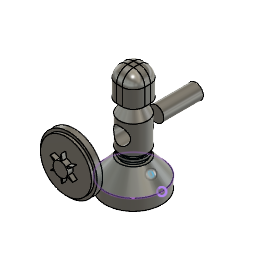
chess- pawn (Autodesk Fusion 360 design; units mm, degrees)
part number: 2026-07-03-03-44-02-403
Autodesk Fusion 360 part; units mm, degrees
sketch "Sketch1" plane through (0, 0, 0) normal (0, 0, 1) x (1, 0, 0)
  line L0 (0, 0) -> (12.7, 0)
  line L1 (12.7, 0) -> (12.7, 5.08)
  line L2 (12.7, 5.08) -> (6.35, 12.8383)
  line L3 (6.35, 12.8383) -> (5.08, 12.8383)
  line L4 (5.08, 12.8383) -> (5.08, 14.1186)
  line L5 (5.08, 14.1186) -> (5.715, 14.1186)
  line L6 (5.715, 14.1186) -> (5.715, 15.24)
  line L7 (5.715, 15.24) -> (5.08, 15.24)
  line L8 (5.08, 15.24) -> (5.08, 16.7432)
  line L9 (5.08, 16.7432) -> (6.35, 16.7432)
  line L10 (6.35, 16.7432) -> (6.35, 29.4432)
  line L11 (6.35, 29.4432) -> (2.54, 35.56)
  line L12 (2.54, 35.56) -> (0, 35.56)
  line L13 (0, 35.56) -> (0, 0)
  dimension "d1" = 12.7
  constraint coincident L0.start L13.end
  constraint horizontal L0
  constraint perpendicular L0 L1
  constraint perpendicular L1 L3
  constraint perpendicular L3 L4
  constraint perpendicular L4 L5
  constraint perpendicular L3 L6
  constraint perpendicular L6 L7
  constraint perpendicular L7 L8
  constraint perpendicular L8 L9
  constraint perpendicular L9 L10
  constraint perpendicular L10 L12
  constraint perpendicular L0 L13
  measures "d1" distance of L9.end L10.end
revolve "Revolve1" add sketch "Sketch1" angle 360 about axis through (0, 35.56, 0) along (0, -1, 0) makes body 1
sketch "Sketch2" plane through (0, 0, 0) normal (0, 0, 1) x (1, 0, 0)
ref_plane "WorkPlane1" through (0, 0, 7.62) normal (0, 0, 1) x (1, 0, 0)
sketch "Sketch3" plane through (0, 0, 7.62) normal (0, 0, 1) x (1, 0, 0)
  circle A0 centre (38.7313, 11.9967) radius 12.7
  dimension "d4" = 25.4
  measures "d4" diameter of A0
extrude "Extrude1" add sketch "Sketch3" along normal blind 2.54 separate body makes body 2
sketch "Sketch4" plane through (0, 0, 10.16) normal (0, 0, 1) x (1, 0, 0)
  circle A0 centre (38.7313, 11.9967) radius 12.7
  circle A1 centre (38.7313, 11.9967) radius 11.43
  dimension "d7" = 22.86
  constraint concentric A0 A1
  measures "d7" diameter of A1
extrude "Extrude2" add sketch "Sketch4" along normal blind 1.27 contours A1 bodies 2
sketch "Sketch5" plane through (0, 0, 11.43) normal (0, 0, 1) x (1, 0, 0)
  circle A0 centre (38.7313, 11.9967) radius 11.43
  circle A1 centre (38.7313, 11.9967) radius 3.2108
  line L0 (37.976, 15.1174) -> (38.638, 17.1526)
  line L1 (38.638, 17.1526) -> (39.2641, 15.163)
  constraint concentric A0 A1
  constraint coincident A1 L0.start
  constraint coincident A1 L1.end
extrude "Extrude3" add sketch "Sketch5" along normal blind 2.54 contours A1 bodies 2
sketch "Sketch6" plane through (0, 0, 11.43) normal (0, 0, 1) x (1, 0, 0)
  circle A0 centre (38.7313, 11.9967) radius 3.2108
  circle A1 centre (38.7313, 11.9967) radius 11.43
  line L0 (38.1005, 15.145) -> (38.5764, 17.7658)
  line L1 (38.5764, 17.7658) -> (39.0696, 15.1896)
  arc A2 (39.0696, 15.1896) -> (38.1005, 15.145) centre (38.7313, 11.9967) ccw
  constraint coincident A0 L0.start
  constraint coincident A0 L1.end
extrude "Extrude4" add sketch "Sketch6" along normal blind 2.032 contours A0 L0 L1 A2 bodies 2
pattern_circular "C-Pattern1" count 6 over 360 about axis through (38.7313, 11.9967, 13.97) along (0, 0, 1) of "Extrude4"
hole "Hole1" at (0, 23.5919, 6.35) direction (0, 0, -1) diameter 7.62 depth 12.7 tip angle 118 bodies 1
sketch "Sketch7" plane through (0, 0, 7.62) normal (0, 0, -1) x (-1, 0, 0)
  circle A0 centre (-38.7313, 11.9967) radius 12.7
  circle A1 centre (-38.7313, 11.9967) radius 3.429
  dimension "d19" = 6.858
  constraint concentric A0 A1
  measures "d19" diameter of A1
extrude "Extrude5" cut sketch "Sketch7" against normal blind 3.048 contours A1 bodies 2
sketch "Sketch8" plane through (0, 0, 0) normal (0, 0, 1) x (1, 0, 0)
  circle A0 centre (-25.4, 12.7) radius 3.429
  dimension "d22" = 6.858
  measures "d22" diameter of A0
extrude "Extrude6" add sketch "Sketch8" along normal blind 12.7 separate body makes body 3
move_body "Move1" bodies 3 to x (1, 0, 0) y (0, 1, 0) z (0, 0, 1) at (25.4, 11.176, -5.08)
move_body "Move2" bodies 2 to x (1, 0, 0) y (0, 1, 0) z (0, 0, 1) at (-42.418, 10.668, 1.27)
move_body "Move3" bodies 2 to x (1, 0, 0) y (0, 1, 0) z (0, 0, 1) at (2.54, 0, 0)
move_body "Move4" bodies 2 to x (1, 0, 0) y (0, 1, 0) z (0, 0, 1) at (0, 0, 6.35)
extrude "Extrude7" add 1 faces at (-1.1987, 24.3974, 7.62) along direction (0, 0, 1) blind 5.08 on bodies 3 bodies 3
move_body "Move5" bodies 2 to x (1, 0, 0) y (0, 1, 0) z (0, 0, 1) at (0, 0, -2.54)
shell "Shell1" thickness 0.762 removed faces 0 bodies 2
sketch "Sketch9" plane through (0, 0, 0) normal (0, 0, 1) x (1, 0, 0)
  line L0 (25.4, 25.4) -> (38.1, 25.4)
  line L1 (38.1, 25.4) -> (38.1, 12.7)
  line L2 (38.1, 12.7) -> (25.4, 12.7)
  line L3 (25.4, 12.7) -> (25.4, 25.4)
  constraint horizontal L0
  constraint vertical L1
  constraint horizontal L2
  constraint vertical L3
extrude "Extrude8" add sketch "Sketch9" along normal blind 12.7 separate body makes body 4
fillet "Fillet1" radius 5.08 8 edges at (31.75, 25.4, 12.7) (38.1, 25.4, 6.35) (31.75, 25.4, 0) (25.4, 25.4, 6.35) (38.1, 19.05, 12.7) (38.1, 19.05, 0) (25.4, 19.05, 12.7) (25.4, 19.05, 0) on bodies 4
move_body "Move6" bodies 4 to x (1, 0, 0) y (0, 1, 0) z (0, 0, 1) at (-30.48, 22.86, -5.08)
move_body "Move7" bodies 4 to x (1, 0, 0) y (0, 1, 0) z (0, 0, 1) at (-2.54, 0, 0)
move_body "Move8" bodies 4 to x (1, 0, 0) y (0, 1, 0) z (0, 0, 1) at (1.27, 0, -1.27)
sketch "Sketch10" plane through (0, 0, 0) normal (0, 0, 1) x (1, 0, 0)
  spline S0 degree 3 poles (12.7, 5.08, 0) (12.6903, 5.08, 1.7214) (12.3451, 5.08, 3.4429) (11.664, 5.08, 5.0242) (10.4702, 5.08, 7.7955) (8.2541, 5.08, 10.1126) (5.5386, 5.08, 11.4286) (2.8377, 5.08, 12.7376) (-0.3346, 5.08, 13.0456) (-3.2369, 5.08, 12.2806) (-6.152, 5.08, 11.5122) (-8.7704, 5.08, 9.6674) (-10.475, 5.08, 7.1808) (-11.9134, 5.08, 5.0825) (-12.7, 5.08, 2.544) (-12.7, 5.08, 0) (-12.7, 5.08, -2.9938) (-11.5995, 5.08, -5.9753) (-9.6545, 5.08, -8.2512) (-7.6931, 5.08, -10.5461) (-4.8887, 5.08, -12.1039) (-1.9039, 5.08, -12.5565) (1.0721, 5.08, -13.0077) (4.2026, 5.08, -12.3567) (6.752, 5.08, -10.7564) (9.2949, 5.08, -9.1602) (11.2388, 5.08, -6.6328) (12.129, 5.08, -3.7654) (12.5068, 5.08, -2.5483) (12.6935, 5.08, -1.2742) (12.7, 5.08, 0) knots 0.00002549 0.00002549 0.00002549 0.00002549 0.40672459 0.40672459 0.40672459 1.11952072 1.11952072 1.11952072 1.82851097 1.82851097 1.82851097 2.54064984 2.54064984 2.54064984 3.14159265 3.14159265 3.14159265 3.84877844 3.84877844 3.84877844 4.56190601 4.56190601 4.56190601 5.27293712 5.27293712 5.27293712 5.98217373 5.98217373 5.98217373 6.2832108 6.2832108 6.2832108 6.2832108
  circle A0 centre (7.8435, 9.4354) radius 1.0338
sketch "Sketch11" plane through (0, 0, 0) normal (1, 0, 0) x (0, 0, -1)
move_body "Move9" bodies 4 to x (1, 0, 0) y (0, 1, 0) z (0, 0, 1) at (38.1, 0, 0)
sketch "Sketch12" plane through (0, 35.56, 0) normal (0, -1, 0) x (1, 0, 0)
  arc A0 (44.45, 1.27) -> (39.37, 6.35) centre (39.37, 1.27) ccw
  line L0 (39.37, 6.35) -> (36.83, 6.35)
  arc A1 (36.83, 6.35) -> (31.75, 1.27) centre (36.83, 1.27) ccw
  line L1 (31.75, 1.27) -> (31.75, -1.27)
  arc A2 (31.75, -1.27) -> (36.83, -6.35) centre (36.83, -1.27) ccw
  line L2 (36.83, -6.35) -> (39.37, -6.35)
  arc A3 (39.37, -6.35) -> (44.45, -1.27) centre (39.37, -1.27) ccw
  line L3 (44.45, -1.27) -> (44.45, 1.27)
  line L4 (35.8643, -6.2574) -> (40.3026, -6.2574)
  line L5 (40.3026, -6.2574) -> (40.3026, -4.8621)
  line L6 (40.3026, -4.8621) -> (35.8643, -4.8621)
  line L7 (35.8643, -4.8621) -> (35.8643, -6.2574)
  constraint horizontal L4
  constraint vertical L5
  constraint horizontal L6
  constraint vertical L7
  constraint coincident A2 L4.start
move_body "Move10" bodies 4 to x (1, 0, 0) y (0, 1, 0) z (0, 0, 1) at (-38.1, 0, 0)
move_body "Move11" bodies 3 to x (1, 0, 0) y (0, 1, 0) z (0, 0, 1) at (0, 0, -22.86)
move_body "Move12" bodies 2 to x (1, 0, 0) y (0, 1, 0) z (0, 0, 1) at (0, 0, 10.16)
move_body "Move13" bodies 2 to x (1, 0, 0) y (0, 1, 0) z (0, 0, 1) at (0, 0, -15.24)
move_body "Move14" bodies 3 to x (1, 0, 0) y (0, 1, 0) z (0, 0, 1) at (0, 0, 20.32)
move_body "Move15" bodies 2 to x (1, 0, 0) y (0, 1, 0) z (0, 0, 1) at (0, 0, 17.78)
move_body "Move16" bodies 3 to x (1, 0, 0) y (0, 1, 0) z (0, 0, 1) at (0, 0, -20.32)
named bodies: "sheild", "pin", "head"
